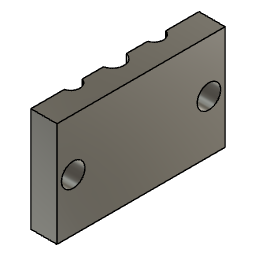
CAD_File 18 (Autodesk Fusion 360 design; units mm, degrees)
Autodesk Fusion 360 part; units mm, degrees
note: some values were not read from the file. Chosen so that the rebuilt part matches the saved one: which bodies a step acts on.
sketch "Sketch1" plane through (0, 0, 0) normal (0, 0, 1) x (1, 0, 0)
  line L0 (5.5, -16.1) -> (-5.5, -16.1)
  line L1 (-5.5, -16.1) -> (-5.5, 16.1)
  line L2 (-5.5, 16.1) -> (5.5, 16.1)
  line L3 (5.5, 16.1) -> (5.5, -16.1)
  line L4 (5.5, -16.1) -> (-5.5, 16.1) construction
  line L5 (-5.5, -16.1) -> (5.5, 16.1) construction
  circle A0 centre (0, 0) radius 2.25
  circle A1 centre (0, 8) radius 1.8
  circle A2 centre (0, -8) radius 1.8
  dimension "d1" = 11
  dimension "d2" = 32.2
  dimension "d3" = 4.5
  dimension "d4" = 3.6
  dimension "d5" = 3.6
  constraint horizontal L0
  constraint perpendicular L0 L1
  constraint parallel L0 L2
  constraint parallel L1 L3
  constraint coincident L4 A0.centre
  constraint coincident L5 A0.centre
  constraint coincident A0.centre origin
  measures "d1" distance of L1.end L2.end
  measures "d2" distance of L0.end L1.end
  measures "d3" diameter of A0
  measures "d4" diameter of A1
  measures "d5" diameter of A2
extrude "Extrude1" add sketch "Sketch1" along normal blind 20 makes body 1
sketch "Sketch2" plane through (0, 0, 20) normal (0, 0, 1) x (-1, 0, 0)
  circle A0 centre (0, 0) radius 2.25
  circle A1 centre (0, 8) radius 1.8
  circle A2 centre (0, -8) radius 1.8
  line L0 (-5.5, -16.1) -> (5.5, -16.1)
  line L1 (5.5, -16.1) -> (5.5, 16.1)
  line L2 (5.5, 16.1) -> (-5.5, 16.1)
  line L3 (-5.5, 16.1) -> (-5.5, -16.1)
  line L4 (-0.5, 16.1) -> (0.5, 16.1)
  line L5 (0.5, 16.1) -> (0.5, -16.1)
  line L6 (0.5, -16.1) -> (-0.5, -16.1)
  line L7 (-0.5, -16.1) -> (-0.5, 16.1)
  line L8 (-0.5, 16.1) -> (0.5, -16.1) construction
  line L9 (0.5, 16.1) -> (-0.5, -16.1) construction
  dimension "d8" = 1
  dimension "d9" = 32.2
  constraint horizontal L4
  constraint perpendicular L4 L5
  constraint parallel L4 L6
  constraint parallel L5 L7
  constraint coincident L8 A0.centre
  constraint coincident L9 A0.centre
  constraint coincident A0.centre origin
  measures "d8" distance of L5.end L6.end
  measures "d9" distance of L4.end L5.end
extrude "Extrude2" cut sketch "Sketch2" against normal blind 20 contours A0 A1 L5 L7 | A0 A2 L5 L7 | A1 L2 L4 L5 L7 | A2 L0 L5 L6 L7 bodies 1 makes body 2 at (5.5, 5.3667, 6.6667)
sketch "Sketch3" plane through (5.5, 0, 0) normal (1, 0, 0) x (0, 1, 0)
  line L0 (-16.1, 0) -> (16.1, 0)
  line L1 (16.1, 0) -> (16.1, 20)
  line L2 (16.1, 20) -> (-16.1, 20)
  line L3 (-16.1, 20) -> (-16.1, 0)
  circle A0 centre (13, 10) radius 2.25
  circle A1 centre (-13, 10) radius 2.25
  dimension "d12" = 4.5
  dimension "d13" = 4.5
  measures "d12" diameter of A0
  measures "d13" diameter of A1
extrude "Extrude3" cut sketch "Sketch3" against normal blind 11 contours A0 | A1 bodies 1 2
delete_body "RemoveBody1" bodies 1
